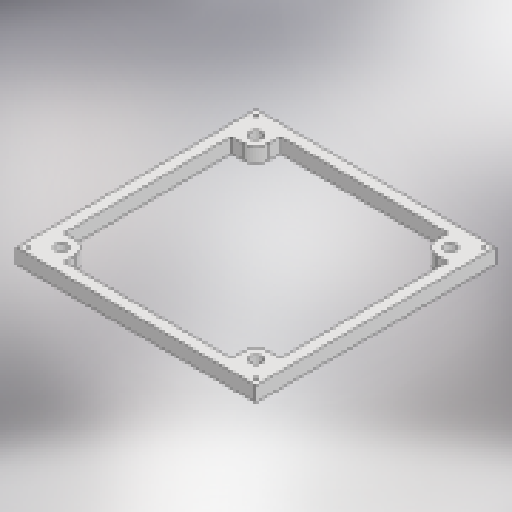
# Autodesk Inventor part: Layer 1
Saved by Autodesk Inventor 2024 (Build 280153000, 153)
## iProperties
Created: 2023-04-21
Part Number: Layer 1
Material: Generic
Document SubType Name: Modeling
Designer: byrne
Density: 1 g/cm^3
Appearance: Default
Author: byrne
Autodesk Inventor part; units mm, degrees
ref_plane "YZ Plane" through (0, 0, 0) normal (1, 0, 0) x (0, 1, 0)
ref_plane "XZ Plane" through (0, 0, 0) normal (0, 1, 0) x (-1, 0, 0)
ref_plane "XY Plane" through (0, 0, 0) normal (0, 0, 1) x (1, 0, 0)
sketch "Sketch1" plane through (0, 0, 0) normal (0, 1, 0) x (-1, 0, 0)
  line L0 (0, 0) -> (101.6, 0)
  line L1 (101.6, 0) -> (101.6, -101.6)
  line L2 (101.6, -101.6) -> (0, -101.6)
  line L3 (0, -101.6) -> (0, 0)
  line L4 (4.7625, -96.8375) -> (96.8375, -96.8375)
  line L5 (96.8375, -96.8375) -> (96.8375, -4.7625)
  line L6 (96.8375, -4.7625) -> (4.7625, -4.7625)
  line L7 (4.7625, -4.7625) -> (4.7625, -96.8375)
  circle A0 centre (9.525, -9.525) radius 2.5527
  circle A1 centre (9.525, -9.525) radius 5.7277
  line L8 (9.525, -15.2527) -> (4.7625, -15.2527)
  line L9 (15.2527, -9.525) -> (15.2527, -4.7625)
  circle A2 centre (9.525, -92.075) radius 2.5527
  circle A3 centre (9.525, -92.075) radius 5.7277
  line L10 (15.2527, -92.075) -> (15.2527, -96.8375)
  line L11 (9.525, -86.3473) -> (4.7625, -86.3473)
  circle A4 centre (92.075, -92.075) radius 2.5527
  circle A5 centre (92.075, -92.075) radius 5.7277
  line L12 (92.075, -86.3473) -> (96.8375, -86.3473)
  line L13 (86.3473, -92.075) -> (86.3473, -96.8375)
  circle A6 centre (92.075, -9.525) radius 2.5527
  circle A7 centre (92.075, -9.525) radius 5.7277
  line L14 (86.3473, -9.525) -> (86.3473, -4.7625)
  line L15 (92.075, -15.2527) -> (96.8375, -15.2527)
  line L16 (57.15, -4.7625) -> (44.45, -4.7625)
  line L17 (44.45, -4.7625) -> (44.45, -34.1313)
  line L18 (44.45, -34.1313) -> (57.15, -34.1313)
  line L19 (57.15, -34.1313) -> (57.15, -4.7625)
  line L20 (57.15, -96.8375) -> (44.45, -96.8375)
  line L21 (44.45, -96.8375) -> (44.45, -57.15)
  line L22 (44.45, -57.15) -> (57.15, -57.15)
  line L23 (57.15, -57.15) -> (57.15, -96.8375)
  line L24 (57.15, -34.1312) -> (44.45, -34.1312)
  line L25 (44.45, -34.1312) -> (44.45, -57.15) construction
  line L26 (44.45, -57.15) -> (57.15, -57.15)
  line L27 (57.15, -57.15) -> (57.15, -34.1312) construction
  point P0 (50.8, -50.8)
  point P1 (0, -50.8)
  point P2 (50.8, 0)
  point P3 (50.8, -4.7625)
  point P4 (50.8, -4.7625)
  point P5 (50.8, -96.8375)
  point P6 (50.8, -96.8375)
  point P7 (50.8, -34.1312)
  point P8 (50.8, -34.1313)
  point P9 (50.8, -50.8)
  point P10 (50.8, -57.15)
  dimension "d0" = 101.6
  dimension "d1" = 101.6
  dimension "d2" = 4.7625
  dimension "d3" = 5.1054
  dimension "d4" = 3.175
  dimension "d5" = 4.7625
  dimension "d6" = 4.7625
  dimension "d9" = 360
  dimension "d13" = 12.7
  dimension "d14" = 39.6875
  dimension "d15" = 29.3687
  dimension "d16" = 12.7
  dimension "d17" = 23.0188
  dimension "d18" = 6.35
  constraints: 56 end point, 10 parallel, 9 midpoint, 8 centre point, 8 point on circle, 7 perpendicular, 5 collinear, 4 coincident, 4 horizontal, 2 point on line, 2 tangent, 2 vertical alignment, 1 horizontal alignment, 40 other
  measures "d0" distance of L1.end L2.end
  measures "d1" distance of L0.end L1.end
  measures "d2" distance between parallel lines of L2 L4
  measures "d3" diameter of A0
  measures "d4" radial gap between concentric circles of A0 A1
  measures "d5" distance from line of L7 A0.centre
  measures "d6" distance from line of L6 A0.centre
  measures "d13" distance of L17.end L18.end
  measures "d14" distance of L22.end L20.start
  measures "d15" distance of L18.end L16.start
  measures "d16" distance between parallel lines of L25 L27
  measures "d17" distance between parallel lines of L26 L24
  measures "d18" distance from line of L26 point (50.8, -50.8)
extrude "Extrusion1" add sketch "Sketch1" along normal blind 6.35 contours L0 L1 L2 L3 | L4 A3 L10 | A3 L4 | L4 A3 L7 | L4 L7 A3 | A3 L7 L11 | L13 A5 L4 | A3 L7 | A5 L5 L4 | L4 A5 | L7 A1 L8 | A5 L5 L4 | L12 L5 A5 | A1 L7 | L7 A1 L6 | L5 A5 | L7 L6 A1 | A1 L6 L9 | L15 A7 L5 | A1 L6 | A7 L6 L5 | L5 A7 | A7 L6 L5 | L14 L6 A7 | L6 A7
sketch "Sketch2" plane through (0, 6.35, 0) normal (0, 1, 0) x (1, 0, 0)
  line L0 (0, 101.6) -> (-101.6, 101.6) projected
  line L1 (-101.6, 101.6) -> (-101.6, 0) projected
  line L2 (-101.6, 0) -> (0, 0) projected
  line L3 (0, 0) -> (0, 101.6) projected
  circle A0 centre (-9.525, 9.525) radius 2.5527 projected
  arc A1 (-9.525, 15.2527) -> (-15.2527, 9.525) centre (-9.525, 9.525) ccw projected
  line L4 (-15.2527, 9.525) -> (-15.2527, 4.7625) projected
  line L5 (-15.2527, 4.7625) -> (-86.3473, 4.7625) projected
  line L6 (-86.3473, 4.7625) -> (-86.3473, 9.525) projected
  arc A2 (-86.3473, 9.525) -> (-92.075, 15.2527) centre (-92.075, 9.525) ccw projected
  line L7 (-92.075, 15.2527) -> (-96.8375, 15.2527) projected
  line L8 (-96.8375, 15.2527) -> (-96.8375, 86.3473) projected
  line L9 (-96.8375, 86.3473) -> (-92.075, 86.3473) projected
  arc A3 (-92.075, 86.3473) -> (-86.3473, 92.075) centre (-92.075, 92.075) ccw projected
  line L10 (-86.3473, 92.075) -> (-86.3473, 96.8375) projected
  line L11 (-86.3473, 96.8375) -> (-15.2527, 96.8375) projected
  line L12 (-15.2527, 96.8375) -> (-15.2527, 92.075) projected
  arc A4 (-15.2527, 92.075) -> (-9.525, 86.3473) centre (-9.525, 92.075) ccw projected
  line L13 (-9.525, 86.3473) -> (-4.7625, 86.3473) projected
  line L14 (-4.7625, 86.3473) -> (-4.7625, 15.2527) projected
  line L15 (-4.7625, 15.2527) -> (-9.525, 15.2527) projected
  circle A5 centre (-9.525, 92.075) radius 2.5527 projected
  circle A6 centre (-92.075, 92.075) radius 2.5527 projected
  circle A7 centre (-92.075, 9.525) radius 2.5527 projected
  circle A8 centre (-99.2188, 99.2188) radius 0.7938
  circle A9 centre (-99.2188, 2.3813) radius 0.7938
  circle A10 centre (-2.3813, 99.2188) radius 0.7938
  circle A11 centre (-2.3813, 2.3813) radius 0.7938
  dimension "d20" = 1.5875
  dimension "d21" = 2.3813
  dimension "d22" = 2.3813
  dimension "d25" = 96.8375
  dimension "d28" = 96.8375
  constraints: 4 centre point, 1 horizontal, 1 vertical, 6 other
  measures "d20" diameter of A8
  measures "d21" distance from line of L0 A8.centre
  measures "d22" distance from line of L1 A8.centre
  measures "d25" distance of A8.centre A9.centre
  measures "d28" distance of A8.centre A10.centre
extrude "Extrusion2" cut sketch "Sketch2" against normal blind 6.35 contours A8 | A9 | A10 | A11
sketch "Sketch3" plane through (0, 6.35, 0) normal (0, 1, 0) x (1, 0, 0)
  circle A0 centre (-99.2188, 99.2188) radius 0.7938 projected
  circle A1 centre (-99.2188, 2.3813) radius 0.7938 projected
  circle A2 centre (-2.3813, 99.2188) radius 0.7938 projected
  circle A3 centre (-2.3813, 2.3813) radius 0.7938 projected
  line L0 (0, 101.6) -> (-101.6, 101.6) projected
  line L1 (-101.6, 101.6) -> (-101.6, 0) projected
  line L2 (-101.6, 0) -> (0, 0) projected
  line L3 (0, 0) -> (0, 101.6) projected
  circle A4 centre (-9.525, 9.525) radius 2.5527 projected
  arc A5 (-9.525, 15.2527) -> (-15.2527, 9.525) centre (-9.525, 9.525) ccw projected
  line L4 (-15.2527, 9.525) -> (-15.2527, 4.7625) projected
  line L5 (-15.2527, 4.7625) -> (-86.3473, 4.7625) projected
  line L6 (-86.3473, 4.7625) -> (-86.3473, 9.525) projected
  arc A6 (-86.3473, 9.525) -> (-92.075, 15.2527) centre (-92.075, 9.525) ccw projected
  line L7 (-92.075, 15.2527) -> (-96.8375, 15.2527) projected
  line L8 (-96.8375, 15.2527) -> (-96.8375, 86.3473) projected
  line L9 (-96.8375, 86.3473) -> (-92.075, 86.3473) projected
  arc A7 (-92.075, 86.3473) -> (-86.3473, 92.075) centre (-92.075, 92.075) ccw projected
  line L10 (-86.3473, 92.075) -> (-86.3473, 96.8375) projected
  line L11 (-86.3473, 96.8375) -> (-15.2527, 96.8375) projected
  line L12 (-15.2527, 96.8375) -> (-15.2527, 92.075) projected
  arc A8 (-15.2527, 92.075) -> (-9.525, 86.3473) centre (-9.525, 92.075) ccw projected
  line L13 (-9.525, 86.3473) -> (-4.7625, 86.3473) projected
  line L14 (-4.7625, 86.3473) -> (-4.7625, 15.2527) projected
  line L15 (-4.7625, 15.2527) -> (-9.525, 15.2527) projected
  circle A9 centre (-9.525, 92.075) radius 2.5527 projected
  circle A10 centre (-92.075, 92.075) radius 2.5527 projected
  circle A11 centre (-92.075, 9.525) radius 2.5527 projected
equation "\"d6\" = d5"
body "Solid1"
